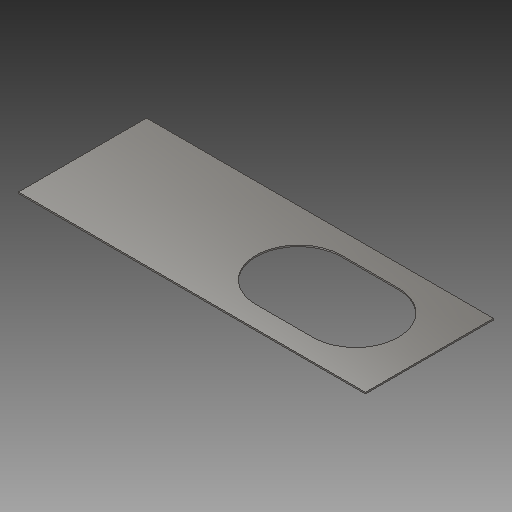
# Autodesk Inventor part: Cabin Roof
Saved by Autodesk Inventor 2019 (Build 230136000, 136)
## iProperties
Created: 2019-08-28
Part Number: Cabin Roof
Material: Steel, Mild
Document SubType Name: Modeling
Designer: DIBYOJYOTI
Density: 7.85 g/cm^3
Appearance: Semi-Polished
Mass: 131.209 g
Surface Area: 343.652 cm^2
Volume: 16.7146 cm^3
Author: DIBYOJYOTI
Autodesk Inventor part; units mm, degrees
ref_plane "YZ Plane" through (0, 0, 0) normal (1, 0, 0) x (0, 1, 0)
ref_plane "XZ Plane" through (0, 0, 0) normal (0, 1, 0) x (-1, 0, 0)
ref_plane "XY Plane" through (0, 0, 0) normal (0, 0, 1) x (1, 0, 0)
sketch "Sketch1" plane through (0, 0, 0) normal (0, 1, 0) x (-1, 0, 0)
  line L0 (-121.9, 45) -> (121.9, 45)
  line L1 (121.9, 45) -> (121.9, -45)
  line L2 (121.9, -45) -> (-121.9, -45)
  line L3 (-121.9, -45) -> (-121.9, 45)
  line L4 (-121.9, 45) -> (121.9, -45) construction
  line L5 (121.9, 45) -> (-121.9, -45) construction
  line L6 (0, 0) -> (-100, 0) construction
  line L7 (-30, 30) -> (-70, 30)
  line L8 (-70, -30) -> (-30, -30)
  arc A0 (-30, -30) -> (-30, 30) centre (-30, 0) ccw
  arc A1 (-70, 30) -> (-70, -30) centre (-70, 0) ccw
  point P0 (-50, 0)
  dimension "d0" = 243.8
  dimension "d1" = 90
  dimension "d2" = 100
  dimension "d4" = 30
  dimension "d5" = 21.9
  constraints: 20 end point, 6 point on circle, 4 tangent, 3 midpoint, 3 parallel, 2 centre point, 2 horizontal, 2 point on line, 1 perpendicular
  measures "d0" distance of L1.end L2.end
  measures "d1" distance of L0.end L1.end
  measures "d2" distance of L6.start L6.end
  measures "d4" radius of A1
  measures "d5" distance from line of L3 L6.end
extrude "Extrusion1" add sketch "Sketch1" along normal blind 1
body "Solid1"
